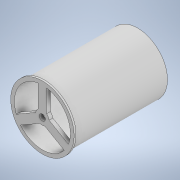
# Autodesk Inventor part: Bobbin-Emma
Saved by Autodesk Inventor 2021 (Build 250183000, 183)
## iProperties
Created: 2023-03-03
Part Number: Bobbin-Emma
Material: Generic
Document SubType Name: Modeling
Designer: egbrown42
Density: 1 g/cm^3
Appearance: Default
Author: egbrown42
Autodesk Inventor part; units mm, degrees
ref_plane "YZ Plane" through (0, 0, 0) normal (1, 0, 0) x (0, 1, 0)
ref_plane "XZ Plane" through (0, 0, 0) normal (0, 1, 0) x (-1, 0, 0)
ref_plane "XY Plane" through (0, 0, 0) normal (0, 0, 1) x (1, 0, 0)
sketch "Sketch1" plane through (0, 0, 0) normal (0, 0, 1) x (1, 0, 0)
  circle A0 centre (0, 0) radius 30
  circle A1 centre (0, 0) radius 32
  dimension "d0" = 60
  dimension "d1" = 2
  constraints: 2 centre point, 2 coincident
  measures "d0" diameter of A0
  measures "d1" radial gap between concentric circles of A0 A1
extrude "Extrusion1" add sketch "Sketch1" along normal blind 100
sketch "Sketch2" plane through (0, 0, 100) normal (0, 0, 1) x (1, 0, 0)
  circle A0 centre (0, 0) radius 34
  circle A1 centre (0, 0) radius 32 projected
  circle A2 centre (0, 0) radius 30 projected
  dimension "d4" = 2
  constraints: 1 centre point, 1 coincident
  measures "d4" radial gap between concentric circles of A1 A0
extrude "Extrusion2" add sketch "Sketch2" along normal blind 2 contours A0 | A1
sketch "Sketch3" plane through (0, 0, 102) normal (0, 0, 1) x (1, 0, 0)
  circle A0 centre (0, 0) radius 3.25
  arc A1 (-4.5086, 5.6776) -> (4.5086, 5.6776) centre (0, 0) ccw
  line L0 (-4.5086, 5.6776) -> (-4.5086, 29.6593)
  circle A2 centre (0, 0) radius 30 projected
  line L1 (4.5086, 5.6776) -> (4.5086, 29.6593)
  dimension "d7" = 6.5
  dimension "d8" = 4
  constraints: 4 end point, 2 centre point, 2 coincident, 2 point on circle, 2 vertical, 2 other
  measures "d7" diameter of A0
  measures "d8" radial gap between concentric circles of A0 A1
extrude "Extrusion3" add sketch "Sketch3" against normal blind 4 contours L0 A2 L1 A1 picked at (0.5026, 13.7724)
pattern_circular "Circular Pattern1" count 3 over 360 about axis through (0, 0, 0) along (0, 0, 1) of "Extrusion3"
body "Solid1"
